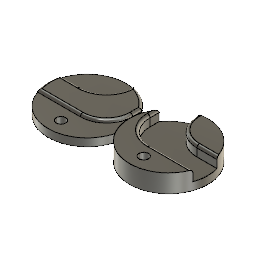
wire_holder v1 (Autodesk Fusion 360 design; units mm, degrees)
Autodesk Fusion 360 part; units mm, degrees
sketch "Sketch1" plane through (0, 0, 0) normal (0, 0, 1) x (1, 0, 0)
  circle A0 centre (0, 0) radius 15
  line L0 (-14.1759, -4.9034) -> (2.2654, -4.9034)
  line L1 (12.2654, 5.0966) -> (12.2654, 8.6348)
  line L2 (-14.4298, 4.0966) -> (-6.7346, 4.0966)
  line L3 (3.2654, 14.0966) -> (3.2654, 14.6403)
  circle A1 centre (-0.2638, -9.8078) radius 1.8
  arc A2 (2.2654, -4.9034) -> (12.2654, 5.0966) centre (2.2654, 5.0966) ccw
  arc A3 (-6.7346, 4.0966) -> (3.2654, 14.0966) centre (-6.7346, 14.0966) ccw
  dimension "d1" = 9
  dimension "d2" = 9
  dimension "d3" = 30
  dimension "d10" = 3.6
  dimension "d19" = 10
  dimension "d22" = 10
  constraint coincident A0.centre origin
  constraint coincident A0 L0.start
  constraint horizontal L0
  constraint perpendicular L0 L1
  constraint coincident A0 L2.start
  constraint horizontal L2
  constraint perpendicular L2 L3
  constraint coincident A0 L1.end
  constraint coincident A0 L3.end
  constraint tangent L0 A2
  constraint tangent L1 A2
  constraint tangent L2 A3
  constraint tangent L3 A3
  measures "d1" distance of L0 L2
  measures "d2" distance of L1 L3
  measures "d3" diameter of A0
  measures "d10" diameter of A1
  measures "d19" radius of A2
  measures "d22" radius of A3
extrude "Extrude1" add sketch "Sketch1" along normal blind 10 contours A0 L0 L1 A2 | A0 L0 L1 L2 L3 A2 A3 | A0 L2 L3 A3 | A1 makes body 1
extrude "Extrude2" cut sketch "Sketch1" along normal blind 7 and the other way blind -3 contours A0 L0 L1 L2 L3 A2 A3 bodies 1
extrude "Extrude3" cut sketch "Sketch1" along normal blind 13 contours A1 bodies 1
fillet "Fillet1" radius 2 1 edges at (-1.942, -9.1569, 10) on bodies 1
split "Split1" by plane through (0, 0, 3) normal (0, 0, 1) bodies 1 makes body 2 at (0.0067, 7.9659, 10)
move_body "Move1" bodies 2 to x (-1, 0, 0) y (0, 1, 0) z (0, 0, -1) at (31.2347, 0, 10)
extrude "Extrude4" add sketch "Sketch1" along normal blind 4 contours A0 L0 L1 L2 L3 A2 A3 bodies 1
fillet "Fillet2" radius 1 1 faces at (-6.215, -1.9034, 4) on bodies 1
fillet "Fillet3" radius 1 5 edges at (41.8168, 4.0966, 7) (27.9692, 14.3684, 7) (37.1899, -4.9034, 7) (21.8982, -1.9745, 7) (18.9692, 6.8657, 7) on bodies 2
